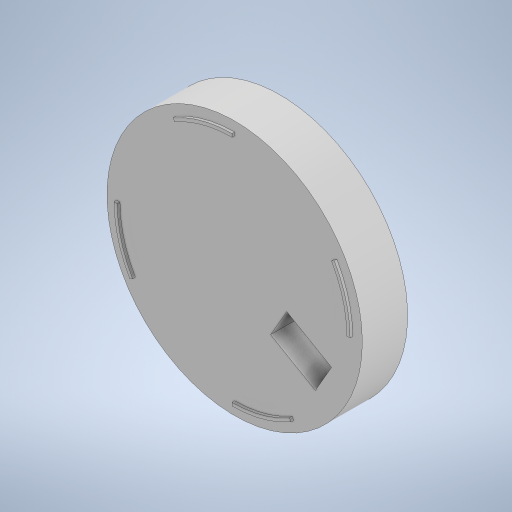
# Autodesk Inventor part: PiezoMount
Saved by Autodesk Inventor 2023 (Build 270158000, 158)
## iProperties
Created: 2023-02-27
Part Number: PiezoMount
Material: Generic
Document SubType Name: Modeling
Designer: maste
Density: 1 g/cm^3
Appearance: Default
Author: maste
Autodesk Inventor part; units mm, degrees
ref_plane "YZ Plane" through (0, 0, 0) normal (1, 0, 0) x (0, 1, 0)
ref_plane "XZ Plane" through (0, 0, 0) normal (0, 1, 0) x (-1, 0, 0)
ref_plane "XY Plane" through (0, 0, 0) normal (0, 0, 1) x (1, 0, 0)
sketch "Sketch1" plane through (0, 0, 0) normal (0, 0, 1) x (1, 0, 0)
  circle A0 centre (0, 0) radius 19.75
  dimension "d2" = 39.5
  constraints: 1 centre point, 1 coincident
  measures "d2" diameter of A0
extrude "Extrusion1" add sketch "Sketch1" along normal blind 1
sketch "Sketch2" plane through (0, 0, 1) normal (0, 0, 1) x (1, 0, 0)
  circle A0 centre (0, 0) radius 17.75
  circle A1 centre (0, 0) radius 18.25
  line L0 (0, 0) -> (18.25, 0)
  arc A2 (18.25, 0) -> (15.805, 9.125) centre (0, 0) ccw
  line L1 (0, 0) -> (15.805, 9.125) construction
  line L2 (0, 0) -> (18.25, 0) construction
  line L3 (15.805, 9.125) -> (15.372, 8.875)
  line L4 (0, 0) -> (0, 18.25)
  line L5 (0, 0) -> (0, -18.25)
  line L6 (0, 0) -> (-18.25, 0)
  line L7 (0, 0) -> (-15.805, -9.125)
  line L8 (0, 0) -> (-9.125, 15.805)
  line L9 (0, 0) -> (9.125, -15.805)
  point P0 (15.805, 9.125)
  point P1 (17.75, 0)
  point P2 (8.875, -15.372)
  point P3 (0, -17.75)
  point P4 (-15.372, -8.875)
  point P5 (-17.75, 0)
  point P6 (-8.875, 15.372)
  point P7 (0, 17.75)
  dimension "d3" = 35.5
  dimension "d4" = 36.5
  dimension "d5" = 30
  constraints: 20 end point, 4 point on line, 3 coincident, 2 perpendicular, 2 point on circle, 1 centre point, 1 horizontal, 1 vertical, 12 other
  measures "d5" angle of L2 L1
extrude "Extrusion2" add sketch "Sketch2" along normal blind 0.4 contours A0 L3 A1 L0 | L9 A1 L5 A0 | A0 L8 A1 L4 | A0 L7 A1 L6
sketch "Sketch3" plane through (0, 0, 1) normal (0, 0, 1) x (1, 0, 0)
  line L0 (0, 0) -> (8.875, -15.372)
  arc A0 (17.75, 0) -> (15.372, 8.875) centre (0, 0) ccw projected
  line L1 (0, 0) -> (17.75, 0)
  arc A1 (0, -17.75) -> (8.875, -15.372) centre (0, 0) ccw projected
  line L2 (8.875, -15.372) -> (17.75, 0)
  line L3 (13.3125, -7.686) -> (0, 0)
  line L4 (13.3125, -7.686) -> (7.2503, -4.186)
  line L5 (12.4955, -10.101) -> (5.5673, -6.101)
  line L6 (5.5673, -6.101) -> (8.0673, -1.7709)
  line L7 (8.0673, -1.7709) -> (14.9955, -5.7709)
  line L8 (14.9955, -5.7709) -> (12.4955, -10.101)
  line L9 (12.4955, -10.101) -> (8.0673, -1.7709) construction
  line L10 (5.5673, -6.101) -> (14.9955, -5.7709) construction
  point P0 (10.2814, -5.936)
  dimension "d13" = 7
  dimension "d14" = 8
  dimension "d15" = 5
  constraints: 22 end point, 4 midpoint, 2 parallel, 1 perpendicular, 1 point on line
  measures "d13" distance of L3.start L4.end
  measures "d14" distance of L5.start L5.end
  measures "d15" distance of L5.end L6.end
extrude "Extrusion3" cut sketch "Sketch3" against normal blind 14 contours L6 L7 L2 L3 | L3 L2 L5 L6 | L2 L7 L8 L5
sketch "Sketch4" plane through (0, 0, 0) normal (0, 0, -1) x (-1, 0, 0)
  line L0 (-12.4955, -10.101) -> (-14.9955, -5.7709) projected
  line L1 (-14.9955, -5.7709) -> (-8.0673, -1.7709) projected
  line L2 (-8.0673, -1.7709) -> (-5.5673, -6.101) projected
  line L3 (-5.5673, -6.101) -> (-12.4955, -10.101) projected
  circle A0 centre (0, 0) radius 19.75 projected
extrude "Extrusion4" add sketch "Sketch4" along normal blind 6
sketch "Sketch5" plane through (0, 0, -6) normal (0, 0, -1) x (-1, 0, 0)
  line L0 (12.5, -12.5) -> (-12.5, -12.5)
  line L1 (-12.5, -12.5) -> (-12.5, 12.5)
  line L2 (-12.5, 12.5) -> (12.5, 12.5)
  line L3 (12.5, 12.5) -> (12.5, -12.5)
  line L4 (12.5, -12.5) -> (-12.5, 12.5) construction
  line L5 (-12.5, -12.5) -> (12.5, 12.5) construction
  point P0 (0, 0)
  dimension "d18" = 25
  dimension "d19" = 25
  constraints: 12 end point, 2 midpoint, 2 parallel, 1 horizontal, 1 perpendicular
  measures "d18" distance of L0.start L0.end
  measures "d19" distance of L0.end L1.end
extrude "Extrusion5" cut sketch "Sketch5" against normal blind 3
sketch "Sketch6" plane through (-12.5, -12.5, -6) normal (1, 0, 0) x (0, 0, -1)
  line L0 (0, 25) -> (0, 0) projected
  line L1 (0, 25) -> (-3, 25) projected
  line L2 (-3, 25) -> (-3, 0) projected
  line L3 (0, 0) -> (-3, 0) projected
  line L4 (-3, 7.5) -> (0, 7.5)
  line L5 (0, 7.5) -> (0, 17.5)
  line L6 (0, 17.5) -> (-3, 17.5)
  line L7 (-3, 17.5) -> (-3, 7.5)
  line L8 (-3, 7.5) -> (0, 17.5) construction
  line L9 (0, 7.5) -> (-3, 17.5) construction
  point P0 (-6, 12.5)
  point P1 (-1.5, 12.5)
  dimension "d22" = 10
  constraints: 12 end point, 2 midpoint, 2 parallel, 1 perpendicular
  measures "d22" distance of L5.end L4.end
extrude "Extrusion6" cut sketch "Sketch6" against normal blind 30 contours L0 L4 L2 L6
body "Solid1"
